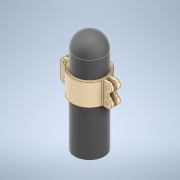
# Autodesk Inventor part: Microscopio
Saved by Autodesk Inventor 2022 (Build 260153000, 153)
## iProperties
Created: 2022-05-08
Part Number: Microscopio
Material: ABS Plastic
Document SubType Name: Modeling
Designer: juanp
Density: 1.06 g/cm^3
Appearance: Smooth - White
Author: juanp
Autodesk Inventor part; units mm, degrees
ref_plane "YZ Plane" through (0, 0, 0) normal (1, 0, 0) x (0, 1, 0)
ref_plane "XZ Plane" through (0, 0, 0) normal (0, 1, 0) x (-1, 0, 0)
ref_plane "XY Plane" through (0, 0, 0) normal (0, 0, 1) x (1, 0, 0)
sketch "Sketch1" plane through (0, 0, 0) normal (0, 1, 0) x (-1, 0, 0)
  circle A0 centre (0, 0) radius 17
  dimension "d0" = 34
  constraints: 1 centre point, 1 coincident
  measures "d0" diameter of A0
extrude "Extrusion1" add sketch "Sketch1" along normal blind 100
sketch "Sketch2" plane through (0, 100, 0) normal (0, 1, 0) x (1, 0, 0)
  circle A0 centre (0, 0) radius 17 projected
  circle A1 centre (0, 0) radius 17 projected
  line L0 (0, -17) -> (0, 17)
  constraints: 2 end point, 2 point on circle, 1 midpoint, 1 vertical
revolve "Revolution1" add sketch "Sketch2" angle 360 about axis through (0, 100, 17) along (0, 0, -1) picked at (5.1055, 2.4587) contours A0 L0
sketch "Sketch3" plane through (0, 0, 0) normal (0, 0, 1) x (1, 0, 0)
  line L0 (20, 54.6) -> (20, 80)
  circle A0 centre (25, 75) radius 1.5
  circle A1 centre (25, 75) radius 5
  circle A2 centre (25, 59.6) radius 1.5
  circle A3 centre (25, 59.6) radius 5
  line L1 (20, 80) -> (25, 80)
  line L2 (20, 54.6) -> (25, 54.6)
  line L3 (28.5355, 63.1355) -> (24.3711, 67.3)
  line L4 (24.3711, 67.3) -> (28.5355, 71.4645)
  line L5 (20, 67.3) -> (24.3711, 67.3) construction
  arc A4 (17, 100) -> (0, 117) centre (0, 100) ccw projected
  arc A5 (0, 117) -> (-17, 100) centre (0, 100) ccw projected
  line L6 (17, 100) -> (17, 0) projected
  line L7 (17, 0) -> (-17, 0) projected
  line L8 (-17, 0) -> (-17, 100) projected
  line L9 (17, 0) -> (17, 100) projected
  line L10 (20, 80) -> (17, 80)
  line L11 (17, 80) -> (17, 54.6)
  line L12 (17, 54.6) -> (20, 54.6)
  line L13 (20, 54.6) -> (20, 80)
  line L14 (0, -24.1042) -> (0, 144.625) projected
  line L15 (28.5355, 78.5355) -> (27.0711, 80)
  line L16 (27.0711, 80) -> (25, 80)
  line L17 (25, 54.6) -> (27.0711, 54.6)
  line L18 (27.0711, 54.6) -> (28.5355, 56.0645)
  point P0 (0, 0)
  point P1 (26.9888, 70.4126)
  point P2 (25.6406, 70.0412)
  point P3 (23.8974, 70.1231)
  point P4 (28.901, 62.7276)
  point P5 (28.7643, 62.8909)
  point P6 (28.7025, 62.9602)
  dimension "d4" = 3
  dimension "d5" = 3.5
  dimension "d6" = 3
  dimension "d7" = 3.5
  dimension "d8" = 45
  dimension "d9" = 25.4
  dimension "d10" = 3
  dimension "d47" = 45
  dimension "d48" = 45
  dimension "d49" = 20
  constraints: 28 end point, 12 point on circle, 8 tangent, 4 centre point, 3 perpendicular, 2 coincident, 2 collinear, 2 parallel, 2 point on line, 1 horizontal, 1 midpoint, 1 vertical
  measures "d4" diameter of A0
  measures "d5" radial gap between concentric circles of A1 A0
  measures "d6" diameter of A2
  measures "d7" radial gap between concentric circles of A3 A2
  measures "d8" angle of L5 L3
  measures "d9" distance between parallel lines of L1 L2
  measures "d10" distance between parallel lines of L0 L6
  measures "d47" angle of L16 L15
  measures "d48" angle of L18 L17
  measures "d49" distance from line of L6.start L10
revolve "Revolution2" add sketch "Sketch3" angle 360 about axis through (0, -10, 0) along (0, 1, 0) separate body contours L12 L6 L10 L0
extrude "Extrusion2" add sketch "Sketch3" along normal blind 4.65 and the other way blind 5.65 contours L12 L6 L10 L0 | L0 A3 L2 | L0 A1 L4 L3 A3 | A3 | A3 L18 L17 | L0 L1 A1 | A1 | L16 L15 A1 bodies 2
extrude "Extrusion3" cut sketch "Sketch3" along normal mid plane 3.3 contours L0 A3 L2 | L0 A1 L4 L3 A3 | A3 | A3 L18 L17 | L0 L1 A1 | A1 | L16 L15 A1 | A0 | A2 bodies 1 2
fillet "Fillet1" radius 2 2 edges at (24.3711, 67.3, 3.15) (24.3711, 67.3, -3.65)
fillet "Fillet2" radius 1.5 2 edges at (19.4519, 67.3, 4.65) (19.1853, 67.3, -5.65)
sketch "Sketch4" plane through (20, 80, 1.65) normal (0, 1, 0) x (1, 0, 0)
  line L0 (0, 3.3) -> (0, 0) projected
  line L1 (0, 0) -> (-68.3024, 0)
  line L2 (-68.3024, 0) -> (-68.3024, 3.3)
  line L3 (-68.3024, 3.3) -> (0, 3.3)
  line L4 (0, 3.3) -> (0, 0)
  line L5 (0, 3.3) -> (7.0711, 3.3) projected
  arc A0 (-1.1383, 8.3012) -> (-0.8357, -4.0709) centre (-20, 1.65) ccw projected
  circle A1 centre (-20, 1.65) radius 17 projected
  point P0 (5, 3.3)
  point P1 (-36.9197, 0)
  point P2 (-36.9197, 3.3)
  point P3 (-39.9318, 3.3)
  point P4 (-39.9318, 0)
  constraints: 8 end point, 2 parallel, 1 collinear, 1 horizontal, 1 perpendicular
extrude "Extrusion4" cut sketch "Sketch4" against normal through all contours A1 L1 A0 L3 bodies 2
sketch "Sketch5" plane through (20, 80, 1.65) normal (0, 1, 0) x (1, 0, 0)
  line L0 (-36.9197, 0) -> (-39.9318, 0) projected
  line L1 (-36.9197, 0) -> (-48.9318, 0)
  line L2 (-48.9318, 0) -> (-48.9318, -3)
  line L3 (-48.9318, -3) -> (-36.9197, -3)
  line L4 (-36.9197, -3) -> (-36.9197, 0)
  circle A0 centre (-20, 1.65) radius 17 projected
  line L5 (-36.9197, 3.3) -> (-48.9318, 3.3)
  line L6 (-48.9318, 3.3) -> (-48.9318, 7.3)
  line L7 (-48.9318, 7.3) -> (-36.9197, 7.3)
  line L8 (-36.9197, 7.3) -> (-36.9197, 3.3)
  dimension "d20" = 3
  dimension "d22" = 9
  dimension "d44" = 4
  constraints: 16 end point, 5 parallel, 2 horizontal, 2 perpendicular, 1 point on circle, 1 point on line
  measures "d20" distance of L1.end L2.end
  measures "d22" distance from line of L2 L0.end
  measures "d44" distance of L5.end L6.end
extrude "Extrusion5" add sketch "Sketch5" against normal up to surface (25.4 mm away) contours L4 L3 L2 L1 L0 | L5 L6 L7 L8 bodies 2
sketch "Sketch6" plane through (-19.1853, 80, -5.65) normal (0, 0, -1) x (-1, 0, 0)
  circle A0 centre (5.2465, -4.5) radius 4.5 construction
  circle A1 centre (5.2465, -20.9) radius 4.5 construction
  line L0 (0, 0) -> (9.7465, 0) construction
  line L1 (9.7465, 0) -> (9.7465, -25.4) construction
  line L2 (0, -25.4) -> (9.7465, -25.4) construction
  circle A2 centre (5.2465, -4.5) radius 1.65
  circle A3 centre (5.2465, -20.9) radius 1.65
  point P0 (-19.1853, -80)
  dimension "d25" = 9
  dimension "d26" = 9
  dimension "d27" = 3.3
  dimension "d28" = 3.3
  constraints: 4 centre point, 4 tangent, 2 coincident
  measures "d25" diameter of A0
  measures "d26" diameter of A1
  measures "d27" diameter of A2
  measures "d28" diameter of A3
extrude "Extrusion6" cut sketch "Sketch6" against normal through all bodies 2
chamfer "Chamfer1" distance 3 angle 45 4 edges at (-28.9318, 80, 3.15) (-28.9318, 80, -3.65) (-28.9318, 54.6, 3.15) (-28.9318, 54.6, -3.65)
sketch "Sketch7" plane through (0, 0, -5.65) normal (0, 0, -1) x (-1, 0, 0)
  line L0 (-20.2763, 80) -> (-20.2763, 54.6) projected
  arc A0 (-28.5355, 78.5355) -> (-28.5355, 71.4645) centre (-25, 75) ccw projected
  line L1 (-28.5355, 71.4645) -> (-25.7853, 68.7142) projected
  arc A1 (-25.7853, 65.8858) -> (-25.7853, 68.7142) centre (-27.1995, 67.3) ccw projected
  line L2 (-25.7853, 65.8858) -> (-28.5355, 63.1355) projected
  arc A2 (-28.5355, 63.1355) -> (-28.5355, 56.0645) centre (-25, 59.6) ccw projected
  circle A3 centre (-25, 59.6) radius 1.5 projected
  circle A4 centre (-25, 75) radius 1.5 projected
  circle A5 centre (24.4318, 59.1) radius 1.65 projected
  circle A6 centre (24.4318, 75.5) radius 1.65 projected
  line L3 (28.9318, 57.6) -> (25.9318, 54.6) projected
  line L4 (28.9318, 77) -> (28.9318, 57.6) projected
  line L5 (25.9318, 80) -> (28.9318, 77) projected
  line L6 (19.1853, 80) -> (25.9318, 80) projected
  line L7 (19.1853, 54.6) -> (19.1853, 80) projected
  line L8 (19.1853, 54.6) -> (25.9318, 54.6) projected
  circle A7 centre (-25, 75) radius 1.5
  line L9 (-28.2447, 75) -> (-26.6224, 77.81)
  line L10 (-26.6224, 77.81) -> (-23.3776, 77.81)
  line L11 (-23.3776, 77.81) -> (-21.7553, 75)
  line L12 (-21.7553, 75) -> (-23.3776, 72.19)
  line L13 (-23.3776, 72.19) -> (-26.6224, 72.19)
  line L14 (-26.6224, 72.19) -> (-28.2447, 75)
  circle A8 centre (-25, 75) radius 5
  line L15 (-28.2447, 75) -> (-30, 75) construction
  circle A9 centre (24.4318, 75.5) radius 1.65
  line L16 (21.1871, 75.5) -> (22.8095, 78.31)
  line L17 (22.8095, 78.31) -> (26.0542, 78.31)
  line L18 (26.0542, 78.31) -> (27.6765, 75.5)
  line L19 (27.6765, 75.5) -> (26.0542, 72.69)
  line L20 (26.0542, 72.69) -> (22.8095, 72.69)
  line L21 (22.8095, 72.69) -> (21.1871, 75.5)
  circle A10 centre (24.4318, 75.5) radius 5
  line L22 (21.1871, 75.5) -> (19.4318, 75.5) construction
  circle A11 centre (24.4318, 59.1) radius 1.65
  line L23 (21.1871, 59.1) -> (22.8095, 61.91)
  line L24 (22.8095, 61.91) -> (26.0542, 61.91)
  line L25 (26.0542, 61.91) -> (27.6765, 59.1)
  line L26 (27.6765, 59.1) -> (26.0542, 56.29)
  line L27 (26.0542, 56.29) -> (22.8095, 56.29)
  line L28 (22.8095, 56.29) -> (21.1871, 59.1)
  circle A12 centre (24.4318, 59.1) radius 5
  line L29 (21.1871, 59.1) -> (19.4318, 59.1) construction
  circle A13 centre (-25, 59.6) radius 1.5
  line L30 (-28.2447, 59.6) -> (-26.6224, 62.41)
  line L31 (-26.6224, 62.41) -> (-23.3776, 62.41)
  line L32 (-23.3776, 62.41) -> (-21.7553, 59.6)
  line L33 (-21.7553, 59.6) -> (-23.3776, 56.79)
  line L34 (-23.3776, 56.79) -> (-26.6224, 56.79)
  line L35 (-26.6224, 56.79) -> (-28.2447, 59.6)
  circle A14 centre (-25, 59.6) radius 5
  line L36 (-28.2447, 59.6) -> (-30, 59.6) construction
  circle A15 centre (-25, 75) radius 1.5 projected
  circle A16 centre (24.4318, 59.1) radius 1.65 projected
  arc A17 (-28.5355, 78.5355) -> (-28.5355, 71.4645) centre (-25, 75) ccw projected
  line L37 (-20.2763, 80) -> (-27.0711, 80) projected
  line L38 (-27.0711, 80) -> (-28.5355, 78.5355) projected
  line L39 (-28.5355, 56.0645) -> (-27.0711, 54.6) projected
  line L40 (-27.0711, 54.6) -> (-20.2763, 54.6) projected
  point P0 (0, 0)
  point P1 (-25, 100)
  dimension "d34" = 5.62
  dimension "d36" = 5.62
  dimension "d38" = 5.62
  dimension "d40" = 5.62
  constraints: 56 end point, 12 coincident, 8 horizontal, 4 centre point, 4 concentric, 4 horizontal alignment, 61 other
  measures "d34" distance between parallel lines of L9 L12
  measures "d36" distance between parallel lines of L16 L19
  measures "d38" distance between parallel lines of L23 L26
  measures "d40" distance between parallel lines of L30 L33
extrude "Extrusion7" cut sketch "Sketch7" against normal blind 2.35 contours L9 L10 L11 L12 L13 L14 | L16 L17 L18 L19 L20 L21 | L23 L24 L25 L26 L27 L28 | L30 L31 L32 L33 L34 L35 bodies 2
body "Solid1"
body "Solid2"
